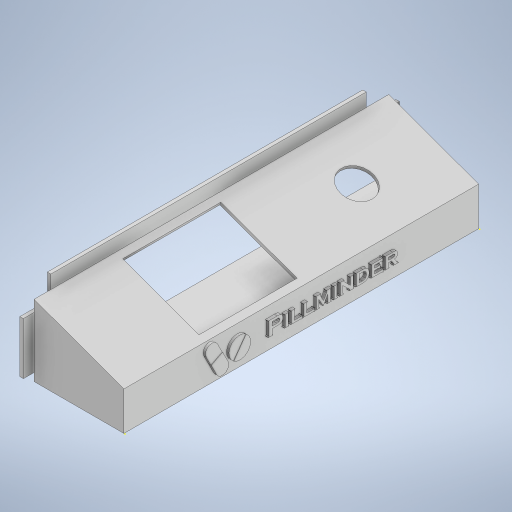
# Autodesk Inventor part: front
Saved by Autodesk Inventor 2024 (Build 280153000, 153)
## iProperties
Created: 2024-01-11
Part Number: front
Material: Generic
Document SubType Name: Modeling
Designer: 96279
Density: 1 g/cm^3
Appearance: Default
Author: 96279
Autodesk Inventor part; units mm, degrees
ref_plane "YZ Plane" through (0, 0, 0) normal (1, 0, 0) x (0, 1, 0)
ref_plane "XZ Plane" through (0, 0, 0) normal (0, 1, 0) x (-1, 0, 0)
ref_plane "XY Plane" through (0, 0, 0) normal (0, 0, 1) x (1, 0, 0)
sketch "Sketch1" plane through (0, 0, 0) normal (0, 1, 0) x (-1, 0, 0)
  line L0 (0.4975, -128.305) -> (38.4975, -128.305)
  line L1 (38.4975, -128.305) -> (38.4975, 21.695)
  line L2 (38.4975, 21.695) -> (0.4975, 21.695)
  line L3 (0.4975, 21.695) -> (0.4975, -128.305)
  line L4 (2.3475, -54.7688) -> (36.6475, -54.7688)
  line L5 (36.6475, -54.7688) -> (36.6475, -13.2688)
  line L6 (36.6475, -13.2688) -> (2.3475, -13.2688)
  line L7 (2.3475, -13.2688) -> (2.3475, -54.7688)
  point P0 (0, 0)
  point P1 (36.583, 517.2316)
  dimension "d0" = 150
  dimension "d5" = 38
  dimension "d23" = 41.5
  dimension "d34" = 1.85
  constraints: 16 end point, 4 parallel, 2 perpendicular, 1 horizontal
  measures "d0" distance of L2.end L0.start
  measures "d5" distance of L1.end L2.end
  measures "d23" distance of L6.end L4.start
  measures "d34" distance between parallel lines of L5 L1
extrude "Extrusion1" add sketch "Sketch1" along normal blind 16.3 contours L3 L2 L1 L0 | L7 L6 L5 L4
sketch "Sketch2" plane through (-0.4975, 0, -128.305) normal (0, 0, -1) x (-1, 0, 0)
  point P0 (-0.4975, 0)
sketch "Sketch4" plane through (-38.4975, 0, -128.305) normal (-1, 0, 0) x (0, 0, 1)
  line L0 (1.5, 15.5) -> (148.5, 15.5)
  line L1 (148.5, 15.5) -> (148.5, 1.5)
  line L2 (148.5, 1.5) -> (1.5, 1.5)
  line L3 (1.5, 1.5) -> (1.5, 15.5)
  line L4 (0, 0) -> (150, 0) projected
  line L5 (0, 0) -> (0, 16.3) projected
  point P0 (-0.3514, 428.1835)
  dimension "d45" = 14
  dimension "d46" = 1.5
  dimension "d47" = 1.5
  dimension "d81" = 147
  constraints: 8 end point, 2 parallel, 1 horizontal, 1 perpendicular
  measures "d45" distance of L2.end L0.start
  measures "d46" distance between parallel lines of L4 L2
  measures "d47" distance between parallel lines of L3 L5
  measures "d81" distance of L0.start L0.end
extrude "Extrusion2" cut sketch "Sketch4" against normal blind 36.5
draft "FaceDraft2" angle 20 pull direction (1, 0, 0) faces at (-13.1642, 16.3, -28.305) fixed edges at (-0.4975, 16.3, -53.305)
draft "FaceDraft3" angle 20 pull direction (-1, 0, 0) faces at (-26.3309, 15.5, -28.805) fixed edges at (-1.9975, 15.5, -53.305)
sketch "Sketch5" plane through (-38.4975, 0, 21.695) normal (0, 0, 1) x (1, 0, 0)
  point P0 (38.4975, 0)
sketch "Sketch6" plane through (-38.4975, 0, -128.305) normal (-1, 0, 0) x (0, 0, 1)
  point P0 (128.305, 0)
sketch "Sketch7" plane through (-38.4975, 0, -128.305) normal (-1, 0, 0) x (0, 0, 1)
  line L0 (148.5, 25.3009) -> (154.5, 25.3009)
  line L1 (154.5, 25.3009) -> (154.5, 3.3009)
  line L2 (154.5, 3.3009) -> (148.5, 3.3009)
  line L3 (148.5, 3.3009) -> (148.5, 25.3009)
  line L4 (-4.5, 25.2907) -> (1.5, 25.2907)
  line L5 (1.5, 25.2907) -> (1.5, 3.2907)
  line L6 (1.5, 3.2907) -> (-4.5, 3.2907)
  line L7 (-4.5, 3.2907) -> (-4.5, 25.2907)
  line L8 (9.525, 35.7976) -> (142.875, 35.7976)
  line L9 (142.875, 35.7976) -> (142.875, 28.7976)
  line L10 (142.875, 28.7976) -> (9.525, 28.7976)
  line L11 (9.525, 28.7976) -> (9.525, 35.7976)
  line L12 (1.5, 28.7849) -> (148.5, 28.7849) projected
  line L13 (1.5, 1.5) -> (1.5, 28.7849) projected
  line L14 (148.5, 28.7849) -> (148.5, 1.5) projected
  point P0 (128.305, 0)
  point P1 (148.5, 25.3009)
  point P2 (148.5, 3.3009)
  point P3 (9.525, 28.7849)
  point P4 (142.875, 28.7849)
  dimension "d52" = 6
  dimension "d53" = 22
  dimension "d54" = 6
  dimension "d55" = 22
  dimension "d56" = 7
  constraints: 24 end point, 6 parallel, 3 horizontal, 3 perpendicular
  measures "d52" distance of L0.start L0.end
  measures "d53" distance of L0.end L1.end
  measures "d54" distance of L4.start L4.end
  measures "d55" distance of L4.end L5.end
  measures "d56" distance of L10.end L8.start
extrude "Extrusion3" add sketch "Sketch7" along normal blind 1.5
sketch "Sketch9" plane through (-0.4975, 16.3, 21.695) normal (0.3420201, 0.9396926, 0) x (0.9396926, -0.3420201, 0)
  line L0 (-3.0698, 76.1079) -> (-37.3698, 76.1079)
  line L1 (-37.3698, 76.1079) -> (-37.3698, 34.6079)
  line L2 (-37.3698, 34.6079) -> (-3.0698, 34.6079)
  line L3 (-3.0698, 34.6079) -> (-3.0698, 76.1079)
  line L4 (-40.4388, 7.125) -> (-40.4388, 0) projected
  line L5 (-40.4388, 140.475) -> (-40.4388, 7.125) projected
  circle A0 centre (-20.2198, 117.475) radius 6.975
  point P0 (6.0425, 21.695)
  dimension "d64" = 41.5
  dimension "d67" = 3.069
  dimension "d68" = 34.3
  dimension "d69" = 13.95
  constraints: 8 end point, 2 parallel, 1 centre point, 1 perpendicular
  measures "d64" distance of L2.end L0.start
  measures "d67" distance between parallel lines of L1 L5
  measures "d68" distance of L0.start L0.end
  measures "d69" diameter of A0
extrude "Extrusion4" cut sketch "Sketch9" against normal blind 1.5
sketch "Sketch10" plane through (-0.4975, 0, 21.695) normal (1, 0, 0) x (0, 0, -1)
  line L0 (59.2774, 12.7341) -> (92.334, 12.7341) construction
  line L1 (92.334, 12.7341) -> (92.334, 5.9901) construction
  line L2 (92.334, 5.9901) -> (59.2774, 5.9901) construction
  line L3 (59.2774, 5.9901) -> (59.2774, 12.7341) construction
  circle A0 centre (47.8893, 8.0599) radius 4.5
  line L4 (45.2768, 4.3959) -> (50.5019, 11.7239)
  line L5 (37.9777, 3.179) -> (33.8075, 11.5176)
  line L6 (38.4727, 14.2287) -> (42.9456, 5.2848)
  arc A1 (37.9777, 3.179) -> (42.9456, 5.2848) centre (40.42, 4.3302) ccw
  arc A2 (38.4727, 14.2287) -> (33.8075, 11.5176) centre (36.194, 12.7805) ccw
  line L7 (40.5577, 10.0597) -> (35.7413, 7.6509)
  line L8 (61.4467, 8.219) -> (61.4467, 6.2089)
  spline S0 degree 2 poles (61.4467, 6.2089) (61.4467, 6.0745) (61.5761, 5.9253) (61.7353, 5.8855) knots 0 0 0 1 2 2 2
  line L9 (61.7353, 5.8855) -> (61.7353, 5.7412)
  line L10 (61.7353, 5.7412) -> (59.8247, 5.7412)
  line L11 (59.8247, 5.7412) -> (59.8247, 5.8855)
  spline S1 degree 2 poles (59.8247, 5.8855) (59.9889, 5.9303) (60.1133, 6.0745) (60.1133, 6.2089) knots 0 0 0 1 2 2 2
  line L12 (60.1133, 6.2089) -> (60.1133, 11.3685)
  spline S2 degree 2 poles (60.1133, 11.3685) (60.1133, 11.5078) (59.9889, 11.6521) (59.8247, 11.6969) knots 0 0 0 1 2 2 2
  line L13 (59.8247, 11.6969) -> (59.8247, 11.8412)
  line L14 (59.8247, 11.8412) -> (63.636, 11.8412)
  spline S3 degree 2 poles (63.636, 11.8412) (64.2977, 11.8412) (65.0838, 11.6621) (65.3824, 11.4431) knots 0 0 0 1 2 2 2
  spline S4 degree 2 poles (65.3824, 11.4431) (65.6909, 11.2143) (65.865, 10.8461) knots 0 0 0 1 1 1
  spline S5 degree 2 poles (65.865, 10.8461) (66.0391, 10.463) (66.0391, 10.0301) knots 0 0 0 1 1 1
  spline S6 degree 2 poles (66.0391, 10.0301) (66.0391, 9.4181) (65.7108, 8.9504) knots 0 0 0 1 1 1
  spline S7 degree 2 poles (65.7108, 8.9504) (65.4222, 8.5524) (64.4818, 8.219) (63.636, 8.219) knots 0 0 0 1 2 2 2
  line L15 (63.636, 8.219) -> (61.4467, 8.219)
  line L16 (61.4467, 9.2241) -> (63.4817, 9.2241)
  spline S8 degree 2 poles (63.4817, 9.2241) (64.0887, 9.2241) (64.3325, 9.3534) knots 0 0 0 1 1 1
  spline S9 degree 2 poles (64.3325, 9.3534) (64.4868, 9.438) (64.6808, 9.8112) (64.6808, 10.0301) knots 0 0 0 1 2 2 2
  spline S10 degree 2 poles (64.6808, 10.0301) (64.6808, 10.249) (64.4868, 10.6222) (64.3325, 10.7068) knots 0 0 0 1 2 2 2
  spline S11 degree 2 poles (64.3325, 10.7068) (64.0887, 10.8361) (63.4817, 10.8361) knots 0 0 0 1 1 1
  line L17 (63.4817, 10.8361) -> (61.4467, 10.8361)
  line L18 (61.4467, 10.8361) -> (61.4467, 9.2241)
  line L19 (68.2085, 10.2938) -> (68.2085, 6.1989)
  spline S12 degree 2 poles (68.2085, 6.1989) (68.2085, 6.0646) (68.3329, 5.9153) (68.4971, 5.8656) knots 0 0 0 1 2 2 2
  line L20 (68.4971, 5.8656) -> (68.4971, 5.7412)
  line L21 (68.4971, 5.7412) -> (66.7208, 5.7412)
  line L22 (66.7208, 5.7412) -> (66.7208, 5.8656)
  spline S13 degree 2 poles (66.7208, 5.8656) (66.88, 5.9054) (67.0094, 6.0596) (67.0094, 6.194) knots 0 0 0 1 2 2 2
  line L23 (67.0094, 6.194) -> (67.0094, 10.2938)
  spline S14 degree 2 poles (67.0094, 10.2938) (67.0094, 10.4281) (66.885, 10.5724) (66.7208, 10.6222) knots 0 0 0 1 2 2 2
  line L24 (66.7208, 10.6222) -> (66.7208, 10.7466)
  line L25 (66.7208, 10.7466) -> (68.4971, 10.7466)
  line L26 (68.4971, 10.7466) -> (68.4971, 10.6222)
  spline S15 degree 2 poles (68.4971, 10.6222) (68.3329, 10.5774) (68.2085, 10.4281) (68.2085, 10.2938) knots 0 0 0 1 2 2 2
  line L27 (70.8604, 6.6467) -> (73.6666, 6.6467)
  spline S16 degree 2 poles (73.6666, 6.6467) (73.8059, 6.6467) (73.9502, 6.7711) (74, 6.9353) knots 0 0 0 1 2 2 2
  line L28 (74, 6.9353) -> (74.1194, 6.9353)
  line L29 (74.1194, 6.9353) -> (74.1194, 5.4526)
  line L30 (74.1194, 5.4526) -> (74, 5.4526)
  spline S17 degree 2 poles (74, 5.4526) (73.9552, 5.6168) (73.8059, 5.7412) (73.6666, 5.7412) knots 0 0 0 1 2 2 2
  line L31 (73.6666, 5.7412) -> (69.3727, 5.7412)
  line L32 (69.3727, 5.7412) -> (69.3727, 5.8656)
  spline S18 degree 2 poles (69.3727, 5.8656) (69.532, 5.9054) (69.6613, 6.0596) (69.6613, 6.194) knots 0 0 0 1 2 2 2
  line L33 (69.6613, 6.194) -> (69.6613, 10.2938)
  spline S19 degree 2 poles (69.6613, 10.2938) (69.6613, 10.4281) (69.5369, 10.5724) (69.3727, 10.6222) knots 0 0 0 1 2 2 2
  line L34 (69.3727, 10.6222) -> (69.3727, 10.7466)
  line L35 (69.3727, 10.7466) -> (71.149, 10.7466)
  line L36 (71.149, 10.7466) -> (71.149, 10.6222)
  spline S20 degree 2 poles (71.149, 10.6222) (70.9848, 10.5774) (70.8604, 10.4281) (70.8604, 10.2888) knots 0 0 0 1 2 2 2
  line L37 (70.8604, 10.2888) -> (70.8604, 6.6467)
  line L38 (76.1196, 6.6467) -> (78.9258, 6.6467)
  spline S21 degree 2 poles (78.9258, 6.6467) (79.0651, 6.6467) (79.2094, 6.7711) (79.2591, 6.9353) knots 0 0 0 1 2 2 2
  line L39 (79.2591, 6.9353) -> (79.3785, 6.9353)
  line L40 (79.3785, 6.9353) -> (79.3785, 5.4526)
  line L41 (79.3785, 5.4526) -> (79.2591, 5.4526)
  spline S22 degree 2 poles (79.2591, 5.4526) (79.2143, 5.6168) (79.0651, 5.7412) (78.9258, 5.7412) knots 0 0 0 1 2 2 2
  line L42 (78.9258, 5.7412) -> (74.6319, 5.7412)
  line L43 (74.6319, 5.7412) -> (74.6319, 5.8656)
  spline S23 degree 2 poles (74.6319, 5.8656) (74.7911, 5.9054) (74.9205, 6.0596) (74.9205, 6.194) knots 0 0 0 1 2 2 2
  line L44 (74.9205, 6.194) -> (74.9205, 10.2938)
  spline S24 degree 2 poles (74.9205, 10.2938) (74.9205, 10.4281) (74.7961, 10.5724) (74.6319, 10.6222) knots 0 0 0 1 2 2 2
  line L45 (74.6319, 10.6222) -> (74.6319, 10.7466)
  line L46 (74.6319, 10.7466) -> (76.4081, 10.7466)
  line L47 (76.4081, 10.7466) -> (76.4081, 10.6222)
  spline S25 degree 2 poles (76.4081, 10.6222) (76.244, 10.5774) (76.1196, 10.4281) (76.1196, 10.2888) knots 0 0 0 1 2 2 2
  line L48 (76.1196, 10.2888) -> (76.1196, 6.6467)
  line L49 (83.0953, 5.7412) -> (81.2692, 9.03)
  line L50 (81.2692, 9.03) -> (81.2692, 6.1989)
  spline S26 degree 2 poles (81.2692, 6.1989) (81.2692, 6.0596) (81.3936, 5.9153) (81.5578, 5.8656) knots 0 0 0 1 2 2 2
  line L51 (81.5578, 5.8656) -> (81.5578, 5.7412)
  line L52 (81.5578, 5.7412) -> (79.891, 5.7412)
  line L53 (79.891, 5.7412) -> (79.891, 5.8656)
  spline S27 degree 2 poles (79.891, 5.8656) (80.0502, 5.9054) (80.1796, 6.0596) (80.1796, 6.194) knots 0 0 0 1 2 2 2
  line L54 (80.1796, 6.194) -> (80.1796, 10.2938)
  spline S28 degree 2 poles (80.1796, 10.2938) (80.1796, 10.4281) (80.0552, 10.5774) (79.891, 10.6222) knots 0 0 0 1 2 2 2
  line L55 (79.891, 10.6222) -> (79.891, 10.7466)
  line L56 (79.891, 10.7466) -> (82.0056, 10.7466)
  line L57 (82.0056, 10.7466) -> (82.0056, 10.6222)
  spline S29 degree 2 poles (82.0056, 10.6222) (81.7966, 10.5575) (81.7966, 10.3684) knots 0 0 0 1 1 1
  spline S30 degree 2 poles (81.7966, 10.3684) (81.7966, 10.1843) (81.9459, 9.9206) knots 0 0 0 1 1 1
  line L58 (81.9459, 9.9206) -> (83.1948, 7.6617)
  line L59 (83.1948, 7.6617) -> (84.4486, 9.8908)
  spline S31 degree 2 poles (84.4486, 9.8908) (84.6626, 10.244) (84.6626, 10.3883) knots 0 0 0 1 1 1
  spline S32 degree 2 poles (84.6626, 10.3883) (84.6626, 10.5724) (84.4436, 10.6222) knots 0 0 0 1 1 1
  line L60 (84.4436, 10.6222) -> (84.4436, 10.7466)
  line L61 (84.4436, 10.7466) -> (86.5085, 10.7466)
  line L62 (86.5085, 10.7466) -> (86.5085, 10.6222)
  spline S33 degree 2 poles (86.5085, 10.6222) (86.3443, 10.5774) (86.2199, 10.4281) (86.2199, 10.2938) knots 0 0 0 1 2 2 2
  line L63 (86.2199, 10.2938) -> (86.2199, 6.1989)
  spline S34 degree 2 poles (86.2199, 6.1989) (86.2199, 6.0646) (86.3443, 5.9104) (86.5085, 5.8656) knots 0 0 0 1 2 2 2
  line L64 (86.5085, 5.8656) -> (86.5085, 5.7412)
  line L65 (86.5085, 5.7412) -> (84.7322, 5.7412)
  line L66 (84.7322, 5.7412) -> (84.7322, 5.8656)
  spline S35 degree 2 poles (84.7322, 5.8656) (84.8914, 5.9054) (85.0208, 6.0596) (85.0208, 6.194) knots 0 0 0 1 2 2 2
  line L67 (85.0208, 6.194) -> (85.0208, 9.03)
  line L68 (85.0208, 9.03) -> (83.0953, 5.7412)
  line L69 (88.8768, 10.2938) -> (88.8768, 6.1989)
  spline S36 degree 2 poles (88.8768, 6.1989) (88.8768, 6.0646) (89.0012, 5.9153) (89.1654, 5.8656) knots 0 0 0 1 2 2 2
  line L70 (89.1654, 5.8656) -> (89.1654, 5.7412)
  line L71 (89.1654, 5.7412) -> (87.3891, 5.7412)
  line L72 (87.3891, 5.7412) -> (87.3891, 5.8656)
  spline S37 degree 2 poles (87.3891, 5.8656) (87.5484, 5.9054) (87.6777, 6.0596) (87.6777, 6.194) knots 0 0 0 1 2 2 2
  line L73 (87.6777, 6.194) -> (87.6777, 10.2938)
  spline S38 degree 2 poles (87.6777, 10.2938) (87.6777, 10.4281) (87.5533, 10.5724) (87.3891, 10.6222) knots 0 0 0 1 2 2 2
  line L74 (87.3891, 10.6222) -> (87.3891, 10.7466)
  line L75 (87.3891, 10.7466) -> (89.1654, 10.7466)
  line L76 (89.1654, 10.7466) -> (89.1654, 10.6222)
  spline S39 degree 2 poles (89.1654, 10.6222) (89.0012, 10.5774) (88.8768, 10.4281) (88.8768, 10.2938) knots 0 0 0 1 2 2 2
  line L77 (91.4193, 9.04) -> (91.4193, 6.1989)
  spline S40 degree 2 poles (91.4193, 6.1989) (91.4193, 6.0596) (91.5487, 5.9104) (91.7079, 5.8656) knots 0 0 0 1 2 2 2
  line L78 (91.7079, 5.8656) -> (91.7079, 5.7412)
  line L79 (91.7079, 5.7412) -> (90.0411, 5.7412)
  line L80 (90.0411, 5.7412) -> (90.0411, 5.8656)
  spline S41 degree 2 poles (90.0411, 5.8656) (90.2003, 5.9054) (90.3297, 6.0596) (90.3297, 6.194) knots 0 0 0 1 2 2 2
  line L81 (90.3297, 6.194) -> (90.3297, 10.2938)
  spline S42 degree 2 poles (90.3297, 10.2938) (90.3297, 10.4281) (90.2053, 10.5724) (90.0411, 10.6222) knots 0 0 0 1 2 2 2
  line L82 (90.0411, 10.6222) -> (90.0411, 10.7466)
  line L83 (90.0411, 10.7466) -> (91.9666, 10.7466)
  line L84 (91.9666, 10.7466) -> (91.9666, 10.6222)
  spline S43 degree 2 poles (91.9666, 10.6222) (91.7676, 10.5724) (91.7676, 10.448) knots 0 0 0 1 1 1
  spline S44 degree 2 poles (91.7676, 10.448) (91.7676, 10.3386) (91.9119, 10.1993) knots 0 0 0 1 1 1
  line L85 (91.9119, 10.1993) -> (94.5937, 7.5324)
  line L86 (94.5937, 7.5324) -> (94.5937, 10.2938)
  spline S45 degree 2 poles (94.5937, 10.2938) (94.5937, 10.4281) (94.4693, 10.5774) (94.3051, 10.6222) knots 0 0 0 1 2 2 2
  line L87 (94.3051, 10.6222) -> (94.3051, 10.7466)
  line L88 (94.3051, 10.7466) -> (95.9719, 10.7466)
  line L89 (95.9719, 10.7466) -> (95.9719, 10.6222)
  spline S46 degree 2 poles (95.9719, 10.6222) (95.8077, 10.5774) (95.6834, 10.4281) (95.6834, 10.2938) knots 0 0 0 1 2 2 2
  line L90 (95.6834, 10.2938) -> (95.6834, 6.1989)
  spline S47 degree 2 poles (95.6834, 6.1989) (95.6834, 6.0646) (95.8077, 5.9153) (95.9719, 5.8656) knots 0 0 0 1 2 2 2
  line L91 (95.9719, 5.8656) -> (95.9719, 5.7412)
  line L92 (95.9719, 5.7412) -> (94.1758, 5.7412)
  line L93 (94.1758, 5.7412) -> (94.1758, 5.8656)
  spline S48 degree 2 poles (94.1758, 5.8656) (94.3748, 5.9054) (94.3748, 6.0298) knots 0 0 0 1 1 1
  spline S49 degree 2 poles (94.3748, 6.0298) (94.3748, 6.0895) (94.2653, 6.2238) (94.0763, 6.4179) knots 0 0 0 1 2 2 2
  line L94 (94.0763, 6.4179) -> (91.4193, 9.04)
  line L95 (97.1412, 6.194) -> (97.1412, 10.2938)
  spline S50 degree 2 poles (97.1412, 10.2938) (97.1412, 10.4281) (97.0168, 10.5724) (96.8526, 10.6222) knots 0 0 0 1 2 2 2
  line L96 (96.8526, 10.6222) -> (96.8526, 10.7466)
  line L97 (96.8526, 10.7466) -> (99.7882, 10.7466)
  spline S51 degree 2 poles (99.7882, 10.7466) (100.7037, 10.7466) (101.2311, 10.5177) knots 0 0 0 1 1 1
  spline S52 degree 2 poles (101.2311, 10.5177) (101.9774, 10.1993) (102.3008, 9.4529) knots 0 0 0 1 1 1
  spline S53 degree 2 poles (102.3008, 9.4529) (102.5297, 8.9355) (102.5297, 8.2439) knots 0 0 0 1 1 1
  spline S54 degree 2 poles (102.5297, 8.2439) (102.5297, 6.9602) (101.7635, 6.2984) knots 0 0 0 1 1 1
  spline S55 degree 2 poles (101.7635, 6.2984) (101.4201, 6.0049) (100.4847, 5.7412) (99.7882, 5.7412) knots 0 0 0 1 2 2 2
  line L98 (99.7882, 5.7412) -> (96.8526, 5.7412)
  line L99 (96.8526, 5.7412) -> (96.8526, 5.8656)
  spline S56 degree 2 poles (96.8526, 5.8656) (97.0118, 5.9054) (97.1412, 6.0596) (97.1412, 6.194) knots 0 0 0 1 2 2 2
  line L100 (98.3403, 6.6467) -> (99.619, 6.6467)
  spline S57 degree 2 poles (99.619, 6.6467) (100.4997, 6.6467) (100.8977, 7.0498) knots 0 0 0 1 1 1
  spline S58 degree 2 poles (100.8977, 7.0498) (101.3107, 7.4677) (101.3107, 8.2439) knots 0 0 0 1 1 1
  spline S59 degree 2 poles (101.3107, 8.2439) (101.3107, 9.0201) (100.8977, 9.438) knots 0 0 0 1 1 1
  spline S60 degree 2 poles (100.8977, 9.438) (100.6887, 9.647) (100.0817, 9.841) (99.619, 9.841) knots 0 0 0 1 2 2 2
  line L101 (99.619, 9.841) -> (98.3403, 9.841)
  line L102 (98.3403, 9.841) -> (98.3403, 6.6467)
  line L103 (104.7836, 7.8707) -> (104.7836, 6.6467)
  line L104 (104.7836, 6.6467) -> (107.963, 6.6467)
  spline S61 degree 2 poles (107.963, 6.6467) (108.0973, 6.6467) (108.2466, 6.7711) (108.2913, 6.9353) knots 0 0 0 1 2 2 2
  line L105 (108.2913, 6.9353) -> (108.4157, 6.9353)
  line L106 (108.4157, 6.9353) -> (108.4157, 5.4526)
  line L107 (108.4157, 5.4526) -> (108.2913, 5.4526)
  spline S62 degree 2 poles (108.2913, 5.4526) (108.2515, 5.6118) (108.0973, 5.7412) (107.958, 5.7412) knots 0 0 0 1 2 2 2
  line L108 (107.958, 5.7412) -> (103.2959, 5.7412)
  line L109 (103.2959, 5.7412) -> (103.2959, 5.8656)
  spline S63 degree 2 poles (103.2959, 5.8656) (103.4551, 5.9054) (103.5845, 6.0596) (103.5845, 6.194) knots 0 0 0 1 2 2 2
  line L110 (103.5845, 6.194) -> (103.5845, 10.2938)
  spline S64 degree 2 poles (103.5845, 10.2938) (103.5845, 10.4281) (103.4601, 10.5724) (103.2959, 10.6222) knots 0 0 0 1 2 2 2
  line L111 (103.2959, 10.6222) -> (103.2959, 10.7466)
  line L112 (103.2959, 10.7466) -> (107.8236, 10.7466)
  spline S65 degree 2 poles (107.8236, 10.7466) (107.963, 10.7466) (108.1122, 10.871) (108.157, 11.0351) knots 0 0 0 1 2 2 2
  line L113 (108.157, 11.0351) -> (108.2764, 11.0351)
  line L114 (108.2764, 11.0351) -> (108.2764, 9.5524)
  line L115 (108.2764, 9.5524) -> (108.157, 9.5524)
  spline S66 degree 2 poles (108.157, 9.5524) (108.1122, 9.7166) (107.963, 9.841) (107.8236, 9.841) knots 0 0 0 1 2 2 2
  line L116 (107.8236, 9.841) -> (104.7836, 9.841)
  line L117 (104.7836, 9.841) -> (104.7836, 8.7414)
  line L118 (104.7836, 8.7414) -> (106.6743, 8.7414)
  spline S67 degree 2 poles (106.6743, 8.7414) (106.8086, 8.7414) (106.9579, 8.8658) (107.0077, 9.03) knots 0 0 0 1 2 2 2
  line L119 (107.0077, 9.03) -> (107.1271, 9.03)
  line L120 (107.1271, 9.03) -> (107.1271, 7.5821)
  line L121 (107.1271, 7.5821) -> (107.0077, 7.5821)
  spline S68 degree 2 poles (107.0077, 7.5821) (106.9629, 7.7413) (106.8136, 7.8707) (106.6743, 7.8707) knots 0 0 0 1 2 2 2
  line L122 (106.6743, 7.8707) -> (104.7836, 7.8707)
  line L123 (110.6597, 7.8011) -> (110.6597, 6.1989)
  spline S69 degree 2 poles (110.6597, 6.1989) (110.6597, 6.0646) (110.7841, 5.9153) (110.9483, 5.8656) knots 0 0 0 1 2 2 2
  line L124 (110.9483, 5.8656) -> (110.9483, 5.7412)
  line L125 (110.9483, 5.7412) -> (109.172, 5.7412)
  line L126 (109.172, 5.7412) -> (109.172, 5.8656)
  spline S70 degree 2 poles (109.172, 5.8656) (109.3312, 5.9054) (109.4606, 6.0596) (109.4606, 6.194) knots 0 0 0 1 2 2 2
  line L127 (109.4606, 6.194) -> (109.4606, 10.2938)
  spline S71 degree 2 poles (109.4606, 10.2938) (109.4606, 10.4281) (109.3362, 10.5724) (109.172, 10.6222) knots 0 0 0 1 2 2 2
  line L128 (109.172, 10.6222) -> (109.172, 10.7466)
  line L129 (109.172, 10.7466) -> (112.4509, 10.7466)
  spline S72 degree 2 poles (112.4509, 10.7466) (113.0927, 10.7466) (113.7595, 10.6172) (114.0232, 10.448) knots 0 0 0 1 2 2 2
  spline S73 degree 2 poles (114.0232, 10.448) (114.5655, 10.0948) (114.5655, 9.2987) knots 0 0 0 1 1 1
  spline S74 degree 2 poles (114.5655, 9.2987) (114.5655, 8.6917) (113.8988, 8.0051) (113.1574, 7.8558) knots 0 0 0 1 2 2 2
  line L130 (113.1574, 7.8558) -> (114.1028, 6.5323)
  spline S75 degree 2 poles (114.1028, 6.5323) (114.3665, 6.1641) (114.675, 5.9004) (114.869, 5.8656) knots 0 0 0 1 2 2 2
  line L131 (114.869, 5.8656) -> (114.869, 5.7412)
  line L132 (114.869, 5.7412) -> (112.7693, 5.7412)
  line L133 (112.7693, 5.7412) -> (112.7693, 5.8656)
  spline S76 degree 2 poles (112.7693, 5.8656) (112.9982, 5.9303) (112.9982, 6.0646) knots 0 0 0 1 1 1
  spline S77 degree 2 poles (112.9982, 6.0646) (112.9982, 6.1641) (112.8539, 6.3681) knots 0 0 0 1 1 1
  line L134 (112.8539, 6.3681) -> (111.8588, 7.8011)
  line L135 (111.8588, 7.8011) -> (110.6597, 7.8011)
  line L136 (110.6597, 8.7066) -> (112.4608, 8.7066)
  spline S78 degree 2 poles (112.4608, 8.7066) (112.8738, 8.7066) (113.0679, 8.7962) knots 0 0 0 1 1 1
  spline S79 degree 2 poles (113.0679, 8.7962) (113.3465, 8.9156) (113.3465, 9.2738) knots 0 0 0 1 1 1
  spline S80 degree 2 poles (113.3465, 9.2738) (113.3465, 9.5922) (112.9584, 9.841) (112.4608, 9.841) knots 0 0 0 1 2 2 2
  line L137 (112.4608, 9.841) -> (110.6597, 9.841)
  line L138 (110.6597, 9.841) -> (110.6597, 8.7066)
  point P0 (21.695, 0)
  point P1 (50.5019, 11.7239)
  point P2 (45.2768, 4.3959)
  constraints: 8 end point, 4 point on circle, 3 centre point, 2 point on line, 1 parallel, 1 perpendicular, 2 other
extrude "Extrusion5" add sketch "Sketch10" along normal blind 1.2 contours A0 L4 | L5 L7 L6 A1 | L8 S0 L9 L10 L11 S1 L12 S2 L13 L14 S3 S4 S5 S6 S7 L15 | L19 S12 L20 L21 L22 S13 L23 S14 L24 L25 L26 S15 | L27 S16 L28 L29 L30 S17 L31 L32 S18 L33 S19 L34 L35 L36 S20 L37 | L38 S21 L39 L40 L41 S22 L42 L43 S23 L44 S24 L45 L46 L47 S25 L48 | L49 L50 S26 L51 L52 L53 S27 L54 S28 L55 L56 L57 S29 S30 L58 L59 S31 S32 L60 L61 L62 S33 L63 S34 L64 L65 L66 S35 L67 L68 | L69 S36 L70 L71 L72 S37 L73 S38 L74 L75 L76 S39 | L77 S40 L78 L79 L80 S41 L81 S42 L82 L83 L84 S43 S44 L85 L86 S45 L87 L88 L89 S46 L90 S47 L91 L92 L93 S48 S49 L94 | L95 S50 L96 L97 S51 S52 S53 S54 S55 L98 L99 S56 | L103 L104 S61 L105 L106 L107 S62 L108 L109 S63 L110 S64 L111 L112 S65 L113 L114 L115 S66 L116 L117 L118 S67 L119 L120 L121 S68 L122 | L123 S69 L124 L125 L126 S70 L127 S71 L128 L129 S72 S73 S74 L130 S75 L131 L132 L133 S76 S77 L134 L135 picked at (49.932, 6.8305)
sketch "Sketch11" plane through (-0.4975, 0, 21.695) normal (1, 0, 0) x (0, 0, -1)
  circle A0 centre (47.8778, 8.0433) radius 4.5
  line L0 (45.2652, 4.3793) -> (50.4903, 11.7073)
  line L1 (37.9661, 3.1624) -> (33.7959, 11.501)
  line L2 (38.4611, 14.2121) -> (42.934, 5.2682)
  arc A1 (37.9661, 3.1624) -> (42.934, 5.2682) centre (40.4084, 4.3136) ccw
  arc A2 (38.4611, 14.2121) -> (33.7959, 11.501) centre (36.1824, 12.7639) ccw
  line L3 (40.5461, 10.0431) -> (35.7297, 7.6343)
  point P0 (21.695, 0)
  point P1 (-81.9581, -25.6914)
  point P2 (-61.4723, -14.11)
  point P3 (-66.6973, -21.4379)
  point P4 (45.2652, 4.3793)
  point P5 (50.4903, 11.7073)
  constraints: 8 end point, 4 point on circle, 3 centre point, 2 point on line, 1 parallel, 1 perpendicular
extrude "Extrusion6" add sketch "Sketch11" along normal blind 1 contours L0 A0 | L1 A2 L2 L3 picked at (45.5925, 8.7837)
body "Solid1"
